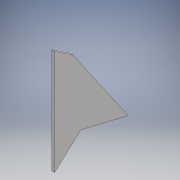
# Autodesk Inventor part: stay_middle
Saved by Autodesk Inventor 2018.1 (Build 221171000, 171)
## iProperties
Created: 2017-10-18
Part Number: stay_middle
Material: 一般
Document SubType Name: Modeling
Designer: kuwano
Density: 1 g/cm^3
Appearance: 既定
Author: kuwano
Autodesk Inventor part; units mm, degrees
ref_plane "YZ Plane" through (0, 0, 0) normal (1, 0, 0) x (0, 1, 0)
ref_plane "XZ Plane" through (0, 0, 0) normal (0, 1, 0) x (-1, 0, 0)
ref_plane "XY Plane" through (0, 0, 0) normal (0, 0, 1) x (1, 0, 0)
sketch "スケッチ1" plane through (0, 0, 0) normal (1, 0, 0) x (0, 1, 0)
  line L0 (-49.976, 100) -> (-49.976, -100)
  line L1 (-49.976, -100) -> (0, -54.2557)
  line L2 (0, -54.2557) -> (90, -75.8767)
  line L3 (-77.9712, 0) -> (117.9952, 0) projected
  line L4 (0, -140) -> (0, 140) projected
  line L5 (-49.976, 100) -> (-15.2492, 76.9448)
  line L6 (-15.2492, 76.9448) -> (90, -75.8767)
  point P0 (0, 0)
  point P1 (-49.976, 0)
  dimension "d0" = 200
  dimension "d1" = 90
  constraints: 10 end point, 2 point on line, 1 midpoint, 1 vertical
  measures "d0" distance of L0.start L0.end
  measures "d1" horizontal distance of L1.end L2.end
extrude "押し出し1" add sketch "スケッチ1" along normal blind 5
